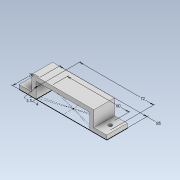
# Autodesk Inventor part: cable_protector
Saved by Autodesk Inventor 2020 (Build 240168000, 168)
## iProperties
Created: 2021-03-03
Part Number: cable_protector
Material: Generic
Document SubType Name: Modeling
Designer: DELL
Density: 1 g/cm^3
Appearance: Default
Author: DELL
Autodesk Inventor part; units mm, degrees
ref_plane "YZ Plane" through (0, 0, 0) normal (1, 0, 0) x (0, 1, 0)
ref_plane "XZ Plane" through (0, 0, 0) normal (0, 1, 0) x (-1, 0, 0)
ref_plane "XY Plane" through (0, 0, 0) normal (0, 0, 1) x (1, 0, 0)
sketch "Sketch1" plane through (0, 0, 0) normal (0, 1, 0) x (-1, 0, 0)
  line L0 (-42.5, -10) -> (42.5, -10)
  line L1 (42.5, -10) -> (42.5, 10)
  line L2 (42.5, 10) -> (-42.5, 10)
  line L3 (-42.5, 10) -> (-42.5, -10)
  line L4 (-42.5, -10) -> (42.5, 10) construction
  line L5 (42.5, -10) -> (-42.5, 10) construction
  line L6 (-30, -10) -> (30, -10)
  line L7 (30, -10) -> (30, 10)
  line L8 (30, 10) -> (-30, 10)
  line L9 (-30, 10) -> (-30, -10)
  line L10 (-30, -10) -> (30, 10) construction
  line L11 (30, -10) -> (-30, 10) construction
  circle A0 centre (36, 0) radius 1.75
  circle A1 centre (-36, 0) radius 1.75
  line L12 (0, 10) -> (0, -10) construction
  line L13 (30, 10) -> (26, 10)
  line L14 (26, 10) -> (26, -10)
  line L15 (26, -10) -> (30, -10)
  line L16 (30, -10) -> (30, 10)
  line L17 (-30, -10) -> (-26, -10)
  line L18 (-26, -10) -> (-26, 10)
  line L19 (-26, 10) -> (-30, 10)
  line L20 (-30, 10) -> (-30, -10)
  point P0 (0, 0)
  point P1 (0, 0)
  dimension "d0" = 72
  dimension "d1" = 60
  dimension "d2" = 85
  dimension "d3" = 3.5
  dimension "d4" = 20
  dimension "d7" = 4
  constraints: 42 end point, 8 parallel, 7 midpoint, 4 horizontal, 4 perpendicular, 3 point on line, 2 centre point, 1 equal radius, 1 horizontal alignment, 1 symmetric about line, 1 other
  measures "d0" distance of A1.centre A0.centre
  measures "d1" distance between parallel lines of L9 L7
  measures "d2" distance between parallel lines of L3 L1
  measures "d3" diameter of A0
  measures "d4" distance between parallel lines of L0 L2
  measures "d7" distance between parallel lines of L7 L14
extrude "Extrusion1" add sketch "Sketch1" along normal blind 4 contours L3 L2 L9 L0 | L7 L2 L1 L0
extrude "Extrusion2" add sketch "Sketch1" along normal blind 15 contours L9 L2 L18 L0 | L14 L2 L7 L0
extrude "Extrusion3" add sketch "Sketch1" along normal blind 4 from surface at 15 contours L9 L2 L18 L0 | L18 L2 L14 L0 | L14 L2 L7 L0
body "Solid1"
